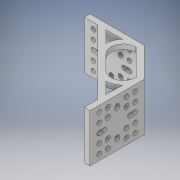
# Autodesk Inventor part: Wheel Corner
Saved by Autodesk Inventor 2019 (Build 230136000, 136)
## iProperties
Created: 2018-12-09
Part Number: Wheel Corner
Material: Generic
Document SubType Name: Modeling
Designer: Ashley
Density: 1 g/cm^3
Appearance: Default
Author: Ashley
Autodesk Inventor part; units mm, degrees
ref_plane "YZ Plane" through (0, 0, 0) normal (1, 0, 0) x (0, 1, 0)
ref_plane "XZ Plane" through (0, 0, 0) normal (0, 1, 0) x (-1, 0, 0)
sketch "Sketch1" plane through (0, 0, 0) normal (0, 1, 0) x (-1, 0, 0)
  line L0 (26.2635, 0) -> (74.2635, 0)
  line L1 (74.2635, 0) -> (74.2635, 5)
  line L2 (5, 74.2635) -> (0, 74.2635)
  line L3 (26.2635, 0) -> (0, 26.2635)
  line L4 (5, 28.3345) -> (28.3345, 5)
  line L5 (0, 74.2635) -> (0, 26.2635)
  line L6 (45.8376, 0) -> (0, 0) construction
  line L7 (0, 0) -> (0, 61.4558) construction
  line L8 (55.1925, 5) -> (5, 55.1925)
  line L9 (5, 62.2635) -> (62.2635, 5)
  line L10 (74.2635, 5) -> (62.2635, 5)
  line L11 (55.1925, 5) -> (28.3345, 5)
  line L12 (5, 28.3345) -> (5, 55.1925)
  line L13 (5, 62.2635) -> (5, 74.2635)
  dimension "d8" = 5
  dimension "d9" = 33
  dimension "d10" = 45
  dimension "d11" = 45
  dimension "d12" = 45.929
  dimension "d13" = 45.929
  dimension "d15" = 0
  dimension "d16" = 135
  dimension "d19" = 45
  dimension "d21" = 135
  dimension "d23" = 5
  dimension "d24" = 12
  dimension "d25" = 12
  dimension "d26" = 5
  dimension "d27" = 5
  dimension "d28" = 5
  dimension "d29" = 5
  dimension "d30" = 45
  dimension "d31" = 45
  dimension "d32" = 135
  dimension "d33" = 135
  dimension "d75" = 48.0001
  constraints: 28 end point, 7 parallel, 4 coincident, 2 horizontal, 1 perpendicular, 1 point on line
  measures "d8" distance between parallel lines of L3 L4
  measures "d9" distance of L4.start L4.end
  measures "d10" angle of L6 L3
  measures "d11" angle of L7 L3
  measures "d12" distance of L1.end L4.end
  measures "d13" distance of L4.start L2.start
  measures "d15" distance between parallel lines of L6 L0
  measures "d16" angle of L0 L3
  measures "d19" angle of L7 L8
  measures "d21" angle of L3 L5
  measures "d23" distance between parallel lines of L9 L8
  measures "d24" distance from line of L2 L9.start
  measures "d25" distance from line of L1 L9.end
  measures "d26" distance between parallel lines of L5 L12
  measures "d27" distance between parallel lines of L5 L13
  measures "d28" distance between parallel lines of L0 L10
  measures "d29" distance between parallel lines of L0 L11
  measures "d30" angle of L11 L8
  measures "d31" angle of L12 L8
  measures "d32" angle of L9 L13
  measures "d33" angle of L4 L12
  measures "d75" distance of L0.start L0.end
extrude "Extrusion1" add sketch "Sketch1" along normal blind 42.7
sketch "Sketch2" plane through (-5, 0, 62.2635) normal (-0.7071068, 0, 0.7071068) x (0.7071068, 0, 0.7071068)
  line L0 (0, 0) -> (-80.9829, 0) construction
  line L1 (0, 0) -> (0, 42.7) construction
  line L2 (-80.9829, 42.7) -> (0, 42.7) construction
  line L3 (-80.9829, 0) -> (-80.9829, 42.7) construction
  line L4 (-75.9829, 0) -> (-75.9829, 42.7) construction
  line L5 (-75.9829, 42.7) -> (-75.9829, 0) construction
  line L6 (-5, 0) -> (-5, 42.7) construction
  line L7 (-75.9829, 0) -> (-5, 0) construction
  line L8 (-5, 42.7) -> (-5, 0) construction
  line L9 (-5, 38.35) -> (-75.9829, 38.35)
  line L10 (-75.9829, 38.35) -> (-75.9829, 4.35)
  line L11 (-75.9829, 4.35) -> (-5, 4.35)
  line L12 (-5, 4.35) -> (-5, 38.35)
  point P0 (-40.4914, 0)
  dimension "d36" = 5
  dimension "d37" = 5
  dimension "d38" = 34
  dimension "d39" = 42.7
  dimension "d40" = 4.35
  dimension "d41" = 4.35
  constraints: 12 end point, 3 equal length, 2 point on line, 1 horizontal, 1 perpendicular, 1 vertical
  measures "d36" distance between parallel lines of L1 L6
  measures "d37" distance between parallel lines of L3 L4
  measures "d38" distance between parallel lines of L11 L9
  measures "d39" distance between parallel lines of L0 L2
  measures "d40" distance between parallel lines of L0 L11
  measures "d41" distance between parallel lines of L2 L9
extrude "Extrusion2" cut sketch "Sketch2" against normal up to surface (5 mm away)
fillet "Fillet1" radius 11 4 edges at (-55.1925, 2.175, 5) (-55.1925, 40.525, 5) (-5, 40.525, 55.1925) (-5, 2.175, 55.1925)
sketch "Sketch3" plane through (0, 42.7, 0) normal (0, 1, 0) x (1, 0, 0)
  arc A0 (-28.6361, -5) -> (-36.4143, -23.7782) centre (-28.6361, -16) ccw construction
  line L0 (-62.2635, -5) -> (-5, -62.2635) construction
  line L1 (0, -74.2635) -> (0, -26.2635) construction
  line L2 (0, -26.2635) -> (-26.2635, 0) construction
  line L3 (-26.2635, 0) -> (-74.2635, 0) construction
  line L4 (-55.1925, -5) -> (-28.6361, -5) construction
  line L5 (-55.1925, -5) -> (-44.6301, -15.5623)
  line L6 (-58.728, -8.5355) -> (-55.1925, -5) construction
  arc A1 (-28.6361, -5) -> (-36.4143, -23.7782) centre (-28.6361, -16) ccw construction
  line L7 (-55.1925, -5) -> (-40.2551, -5)
  arc A2 (-40.2551, -5) -> (-44.6301, -15.5623) centre (-28.6361, -16) ccw
  line L8 (0, 0) -> (-54.4322, -54.4322) construction
  line L9 (-5, -55.1925) -> (-5, -28.3345) construction
  line L10 (-5, -55.1925) -> (-15.5623, -44.6301)
  line L11 (-5, -55.1925) -> (-5, -40.2551)
  arc A3 (-15.5623, -44.6301) -> (-5, -40.2551) centre (-16, -28.6361) ccw
  dimension "d45" = 11
  dimension "d46" = 5
  dimension "d47" = 5
  dimension "d48" = 16
  dimension "d49" = 45
  dimension "d50" = 45
  constraints: 12 end point, 4 point on circle, 4 symmetric about line, 2 centre point, 1 coincident, 1 horizontal, 1 perpendicular, 2 other
  measures "d45" radius of A0
  measures "d46" distance between parallel lines of L0 L5
  measures "d47" distance between parallel lines of L3 L4
  measures "d48" radius of A2
  measures "d49" angle of L1 L8
  measures "d50" angle of L3 L8
extrude "Extrusion3" cut sketch "Sketch3" against normal up to surface (42.7 mm away)
sketch "Sketch5" plane through (-26.2635, 0, 0) normal (0, 0, -1) x (-1, 0, 0)
  line L0 (48.0001, 0) -> (48.0001, 42.7) construction
  line L1 (0, 0) -> (0, 42.7) construction
  line L2 (31.0711, 31.2495) -> (30.5858, 30.7642)
  arc A0 (30.5858, 30.7642) -> (33.4142, 27.9358) centre (32, 29.35) ccw
  line L3 (33.8995, 28.4211) -> (33.4142, 27.9358)
  arc A1 (35.3137, 23.35) -> (35.3137, 19.35) centre (35.3137, 21.35) ccw
  arc A2 (33.8995, 28.4211) -> (31.0711, 31.2495) centre (32.4853, 29.8353) ccw
  line L4 (40, 23.35) -> (35.3137, 23.35)
  circle A3 centre (40, 29.35) radius 2
  arc A4 (40, 19.35) -> (40, 23.35) centre (40, 21.35) ccw
  line L5 (40, 19.35) -> (35.3137, 19.35)
  line L6 (22, 34.0363) -> (22, 32.6637)
  arc A5 (22, 32.6637) -> (26, 32.6637) centre (24, 32.6637) ccw
  line L7 (26, 32.6637) -> (26, 34.0363)
  arc A6 (26, 34.0363) -> (22, 34.0363) centre (24, 34.0363) ccw
  line L8 (8, 19.35) -> (12.6863, 19.35)
  arc A7 (12.6863, 19.35) -> (12.6863, 23.35) centre (12.6863, 21.35) ccw
  line L9 (8, 23.35) -> (12.6863, 23.35)
  arc A8 (8, 23.35) -> (8, 19.35) centre (8, 21.35) ccw
  line L10 (14.1005, 28.4211) -> (14.5858, 27.9358)
  arc A9 (14.5858, 27.9358) -> (17.4142, 30.7642) centre (16, 29.35) ccw
  circle A10 centre (8, 29.35) radius 2
  line L11 (16.9289, 31.2495) -> (17.4142, 30.7642)
  circle A11 centre (8, 37.35) radius 2
  line L12 (16.9289, 35.4505) -> (17.4142, 35.9358)
  line L13 (14.1005, 38.2789) -> (14.5858, 38.7642)
  arc A12 (14.1005, 38.2789) -> (16.9289, 35.4505) centre (15.5147, 36.8647) ccw
  arc A13 (17.4142, 35.9358) -> (14.5858, 38.7642) centre (16, 37.35) ccw
  arc A14 (16.9289, 31.2495) -> (14.1005, 28.4211) centre (15.5147, 29.8353) ccw
  line L14 (33.8995, 14.2789) -> (33.4142, 14.7642)
  arc A15 (33.4142, 14.7642) -> (30.5858, 11.9358) centre (32, 13.35) ccw
  circle A16 centre (40, 13.35) radius 2
  arc A17 (31.0711, 11.4505) -> (33.8995, 14.2789) centre (32.4853, 12.8647) ccw
  line L15 (31.0711, 11.4505) -> (30.5858, 11.9358)
  line L16 (26, 8.6637) -> (26, 10.0363)
  arc A18 (26, 10.0363) -> (22, 10.0363) centre (24, 10.0363) ccw
  line L17 (22, 10.0363) -> (22, 8.6637)
  arc A19 (22, 8.6637) -> (26, 8.6637) centre (24, 8.6637) ccw
  line L18 (31.0711, 7.2495) -> (30.5858, 6.7642)
  arc A20 (33.8995, 4.4211) -> (31.0711, 7.2495) centre (32.4853, 5.8353) ccw
  arc A21 (30.5858, 6.7642) -> (33.4142, 3.9358) centre (32, 5.35) ccw
  circle A22 centre (40, 5.35) radius 2
  line L19 (33.8995, 4.4211) -> (33.4142, 3.9358)
  line L20 (14.1005, 14.2789) -> (14.5858, 14.7642)
  arc A23 (17.4142, 11.9358) -> (14.5858, 14.7642) centre (16, 13.35) ccw
  circle A24 centre (8, 13.35) radius 2
  line L21 (16.9289, 11.4505) -> (17.4142, 11.9358)
  arc A25 (14.1005, 14.2789) -> (16.9289, 11.4505) centre (15.5147, 12.8647) ccw
  line L22 (16.9289, 7.2495) -> (17.4142, 6.7642)
  arc A26 (16.9289, 7.2495) -> (14.1005, 4.4211) centre (15.5147, 5.8353) ccw
  arc A27 (14.5858, 3.9358) -> (17.4142, 6.7642) centre (16, 5.35) ccw
  line L23 (14.1005, 4.4211) -> (14.5858, 3.9358)
  circle A28 centre (8, 5.35) radius 2
  circle A29 centre (40, 37.35) radius 2
  line L24 (31.0711, 35.4505) -> (30.5858, 35.9358)
  arc A30 (31.0711, 35.4505) -> (33.8995, 38.2789) centre (32.4853, 36.8647) ccw
  line L25 (33.8995, 38.2789) -> (33.4142, 38.7642)
  arc A31 (33.4142, 38.7642) -> (30.5858, 35.9358) centre (32, 37.35) ccw
  point P0 (-26.2635, 0)
  dimension "d74" = 48.0001
  dimension "d132" = 42.7
  constraints: 48 end point, 48 point on circle, 32 centre point
  measures "d74" distance between parallel lines of L0 L1
  measures "d132" distance of L0.start L0.end
extrude "Extrusion5" cut sketch "Sketch5" against normal up to surface (5 mm away)
ref_plane "Work Plane1" through (0, 0, 0) normal (-0.7071068, 0, -0.7071068) x (0, 1, 0)
mirror "Mirror1" about plane through (0, 0, 0) normal (-0.7071068, 0, -0.7071068) of "Extrusion5"
sketch "Sketch7" plane through (-5, 0, 28.3345) normal (-0.7071068, 0, 0.7071068) x (0.7071068, 0, 0.7071068)
  circle A0 centre (-16.5, 21.35) radius 5.5
  line L0 (-9.9142, 30.7642) -> (-9.4289, 31.2495)
  arc A1 (-6.6005, 28.4211) -> (-9.4289, 31.2495) centre (-8.0147, 29.8353) ccw
  line L1 (-6.6005, 28.4211) -> (-7.0858, 27.9358)
  arc A2 (-9.9142, 30.7642) -> (-7.0858, 27.9358) centre (-8.5, 29.35) ccw
  arc A3 (-25.9142, 27.9358) -> (-23.0858, 30.7642) centre (-24.5, 29.35) ccw
  line L2 (-25.9142, 27.9358) -> (-26.3995, 28.4211)
  arc A4 (-23.5711, 31.2495) -> (-26.3995, 28.4211) centre (-24.9853, 29.8353) ccw
  line L3 (-23.5711, 31.2495) -> (-23.0858, 30.7642)
  line L4 (-7.0858, 14.7642) -> (-6.6005, 14.2789)
  arc A5 (-9.4289, 11.4505) -> (-6.6005, 14.2789) centre (-8.0147, 12.8647) ccw
  line L5 (-9.4289, 11.4505) -> (-9.9142, 11.9358)
  arc A6 (-7.0858, 14.7642) -> (-9.9142, 11.9358) centre (-8.5, 13.35) ccw
  arc A7 (-23.0858, 11.9358) -> (-25.9142, 14.7642) centre (-24.5, 13.35) ccw
  line L6 (-23.0858, 11.9358) -> (-23.5711, 11.4505)
  arc A8 (-26.3995, 14.2789) -> (-23.5711, 11.4505) centre (-24.9853, 12.8647) ccw
  line L7 (-26.3995, 14.2789) -> (-25.9142, 14.7642)
  line L8 (0, 0) -> (-33, 0) construction
  line L9 (0, 0) -> (0, 42.7) construction
  line L10 (-33, 42.7) -> (0, 42.7) construction
  line L11 (-33, 0) -> (-33, 42.7) construction
  line L12 (-51.9914, 38.35) -> (18.9914, 38.35) construction
  point P0 (-16.5, 0)
  dimension "d144" = 42.7
  dimension "d145" = 33
  dimension "d150" = 8
  dimension "d153" = 17
  dimension "d155" = 8
  dimension "d156" = 8
  dimension "d157" = 8
  dimension "d158" = 8
  dimension "d159" = 8
  dimension "d161" = 8
  dimension "d162" = 8
  dimension "d163" = 11.3137
  dimension "d164" = 33
  dimension "d165" = 16.5
  dimension "d166" = 16.5
  dimension "d167" = 21.35
  constraints: 16 end point, 16 point on circle, 11 centre point
  measures "d144" distance of L8.start L9.end
  measures "d145" distance of L8.start L8.end
  measures "d150" horizontal distance of A3.centre A0.centre
  measures "d153" distance from line of L12 A0.centre
  measures "d155" horizontal distance of A3.centre A0.centre
  measures "d156" horizontal distance of A2.centre A0.centre
  measures "d157" horizontal distance of A2.centre A0.centre
  measures "d158" horizontal distance of A6.centre A0.centre
  measures "d159" horizontal distance of A6.centre A0.centre
  measures "d161" horizontal distance of A7.centre A0.centre
  measures "d162" horizontal distance of A7.centre A0.centre
  measures "d163" distance of A3.centre A0.centre
  measures "d164" distance between parallel lines of L9 L11
  measures "d165" distance from line of L11 A0.centre
  measures "d166" distance from line of L9 A0.centre
  measures "d167" distance from line of L8 A0.centre
extrude "Extrusion7" cut sketch "Sketch7" against normal up to surface (5 mm away)
equation "\"d13\" = d12"
equation "\"d23\" = d8"
equation "\"d25\" = d24"
equation "\"d26\" = d8"
equation "\"d27\" = d8"
equation "\"d28\" = d8"
equation "\"d29\" = d8"
equation "\"d40\" = -0.5 * d38 + 0.5 * d39"
equation "\"d0\" = d8"
equation "\"d1\" = d8"
equation "\"d14\" = d8"
body "Solid1"
